nixal_reprap4040_coil (Autodesk Fusion 360 design; units mm, degrees)
Autodesk Fusion 360 part; units mm, degrees
sketch "Sketch1" plane through (0, 0, 0) normal (0, 1, 0) x (1, 0, 0)
  circle A0 centre (0, 0) radius 5
  circle A1 centre (0, 0) radius 1.7
  circle A2 centre (0, 0) radius 2.75
  circle A3 centre (-3.3842, 0.0229) radius 0.35
  circle A4 centre (-0.0007, -4.252) radius 0.35
  circle A5 centre (0, 0) radius 2.5
  dimension "d1" = 10
  dimension "d2" = 3.4
  dimension "d3" = 5.5
  dimension "d12" = 0.7
  dimension "d13" = 0.7
  dimension "d20" = 5
  constraint coincident A0.centre A1.centre
  constraint concentric A0 A1
  measures "d1" diameter of A0
  measures "d2" diameter of A1
  measures "d3" diameter of A2
  measures "d12" diameter of A3
  measures "d13" diameter of A4
  measures "d20" diameter of A5
extrude "Extrude1" add sketch "Sketch1" along normal blind 12 contours A2 | A5 makes body 1
extrude "Extrude2" add sketch "Sketch1" along normal blind 1 contours A0 | A3 | A4 bodies 1
extrude "Extrude3" add sketch "Sketch1" along normal blind 12 and the other way blind -11 contours A0 | A3 | A4 bodies 1
extrude "Extrude4" [suppressed]
extrude "Extrude5" [suppressed]
extrude "Extrude6" add sketch "Sketch1" along normal blind 14 and the other way blind -12 separate body contours A0 | A2 | A3 makes body 2
